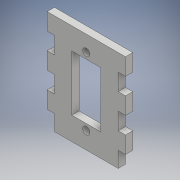
# Autodesk Inventor part: muñeca1
Saved by Autodesk Inventor 2018 (Build 220112000, 112)
## iProperties
Created: 2020-03-11
Part Number: muñeca1
Material: Genérico
Document SubType Name: Modeling
Designer: sala.ceri
Density: 1 g/cm^3
Appearance: Valor por defecto
Author: sala.ceri
Autodesk Inventor part; units mm, degrees
ref_plane "YZ Plane" through (0, 0, 0) normal (1, 0, 0) x (0, 1, 0)
ref_plane "XZ Plane" through (0, 0, 0) normal (0, 1, 0) x (-1, 0, 0)
ref_plane "XY Plane" through (0, 0, 0) normal (0, 0, 1) x (1, 0, 0)
sketch "Boceto1" plane through (0, 0, 0) normal (0, 1, 0) x (-1, 0, 0)
  line L0 (0, 0) -> (26.35, 0)
  line L1 (26.35, 10) -> (0, 10)
  line L2 (26.35, 10) -> (29.35, 10)
  line L3 (29.35, 10) -> (29.35, 0)
  line L4 (29.35, 0) -> (26.35, 0)
  line L5 (0, 10) -> (-3, 10)
  line L6 (-3, 10) -> (-3, 0)
  line L7 (-3, 0) -> (0, 0)
  constraints: 16 end point, 3 horizontal, 3 perpendicular
extrude "Extrusión1" add sketch "Boceto1" along normal blind 3
sketch "Boceto2" plane through (0, 0, 0) normal (0, -1, 0) x (1, 0, 0)
  line L0 (-26.35, 10) -> (-26.35, 40)
  line L1 (-26.35, 47) -> (0, 47)
  line L2 (0, 40) -> (0, 10)
  line L3 (-26.35, 10) -> (0, 10)
  line L4 (-13.175, 15) -> (-7.175, 15)
  line L5 (-7.175, 15) -> (-7.175, 38)
  line L6 (-7.175, 38) -> (-19.175, 38)
  line L7 (-19.175, 38) -> (-19.175, 15)
  line L8 (-19.175, 15) -> (-13.175, 15)
  circle A0 centre (-13.175, 40.5) radius 1.5
  circle A1 centre (-13.175, 12.5) radius 1.5
  line L9 (-26.35, 47) -> (-29.35, 47)
  line L10 (-29.35, 47) -> (-29.35, 40)
  line L11 (-29.35, 40) -> (-26.35, 40)
  line L12 (0, 47) -> (3, 47)
  line L13 (3, 47) -> (3, 40)
  line L14 (3, 40) -> (0, 40)
  point P0 (0, 0)
  dimension "d19" = 7
  dimension "d20" = 3
  constraints: 30 end point, 7 perpendicular, 3 point on line, 2 centre point, 2 horizontal, 2 vertical, 1 parallel
  measures "d19" distance of L9.end L10.end
  measures "d20" distance of L1.end L12.end
extrude "Extrusión2" add sketch "Boceto2" against normal blind 3
sketch "Boceto3" plane through (0, 0, 0) normal (0, -1, 0) x (1, 0, 0)
  line L0 (0, 33) -> (3, 33)
  line L1 (3, 33) -> (3, 26)
  line L2 (3, 26) -> (0, 26)
  line L3 (0, 26) -> (0, 33)
  line L4 (-26.35, 33) -> (-29.35, 33)
  line L5 (-29.35, 33) -> (-29.35, 26)
  line L6 (-29.35, 26) -> (-26.35, 26)
  line L7 (-26.35, 26) -> (-26.35, 33)
  line L8 (-26.35, 19) -> (-29.35, 19)
  line L9 (-29.35, 19) -> (-29.35, 12)
  line L10 (-29.35, 12) -> (-26.35, 12)
  line L11 (-26.35, 12) -> (-26.35, 19)
  line L12 (0, 19) -> (3, 19)
  line L13 (3, 19) -> (3, 12)
  line L14 (3, 12) -> (0, 12)
  line L15 (0, 12) -> (0, 19)
  point P0 (0, 0)
  point P1 (0, 40)
  constraints: 32 end point, 6 perpendicular, 1 horizontal
extrude "Extrusión3" add sketch "Boceto3" against normal blind 3
sketch "Boceto4" plane through (0, 0, 0) normal (0, -1, 0) x (1, 0, 0)
  line L0 (-13.175, 5.5) -> (-26.35, 5.5)
  line L1 (-26.35, 5.5) -> (-29.35, 5.5)
  line L2 (-29.35, 0) -> (-29.35, 10) projected
  line L3 (-13.175, 5.5) -> (3, 5.5)
  line L4 (3, 10) -> (3, 0) projected
  line L5 (3, 0) -> (-29.35, 0) projected
  line L6 (3, 5.5) -> (3, 0)
  line L7 (3, 0) -> (-29.35, 0)
  line L8 (-29.35, 0) -> (-29.35, 5.5)
  point P0 (0, 0)
  point P1 (-13.175, 12.5)
  point P2 (-26.35, 10)
  constraints: 12 end point, 3 point on line, 2 perpendicular, 1 horizontal, 1 vertical
extrude "Extrusión4" cut sketch "Boceto4" against normal blind 3
sketch "Boceto5" plane through (0, 0, 0) normal (0, -1, 0) x (1, 0, 0)
  line L0 (-26.35, 10) -> (-26.35, 12) projected
  line L1 (-26.35, 10) -> (-26.35, 5.5)
  line L2 (-26.35, 5.5) -> (-29.35, 5.5)
  line L3 (-29.35, 10) -> (-26.35, 10) projected
  line L4 (-29.35, 5.5) -> (-29.35, 10)
  line L5 (-29.35, 10) -> (-26.35, 10)
  line L6 (0, 10) -> (3, 10) projected
  line L7 (0, 10) -> (3, 10)
  line L8 (3, 10) -> (3, 5.5) projected
  line L9 (3, 10) -> (3, 5.5)
  line L10 (3, 5.5) -> (0, 5.5)
  line L11 (0, 10) -> (0, 5.5)
  point P0 (0, 0)
  constraints: 16 end point, 3 perpendicular, 2 collinear, 1 horizontal, 1 vertical
extrude "Extrusión5" cut sketch "Boceto5" against normal blind 3
